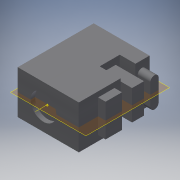
# Autodesk Inventor part: 00_RGB_Laser_Laserlands
Saved by Autodesk Inventor 2019.4 (Build 234330000, 330)
## iProperties
Created: 2021-09-30
Part Number: 00_RGB_Laser_Laserlands
Material: Generic
Document SubType Name: Modeling
Designer: diederichbenedict
Density: 1 g/cm^3
Appearance: Light Gray
Author: diederichbenedict
Autodesk Inventor part; units mm, degrees
ref_plane "YZ Plane" through (0, 0, 0) normal (1, 0, 0) x (0, 1, 0)
ref_plane "XZ Plane" through (0, 0, 0) normal (0, 1, 0) x (-1, 0, 0)
ref_plane "XY Plane" through (0, 0, 0) normal (0, 0, 1) x (1, 0, 0)
sketch "Sketch1" plane through (0, 0, 0) normal (0, 1, 0) x (-1, 0, 0)
  line L0 (0, 0) -> (41, 0)
  line L1 (0, 0) -> (41, 0) construction
  line L2 (41, 0) -> (41, -51)
  line L3 (41, -51) -> (3.5, -51)
  line L4 (3.5, -51) -> (3.5, -41.5)
  line L5 (3.5, -41.5) -> (14, -41.5)
  line L6 (14, -41.5) -> (14, -28)
  line L7 (14, -28) -> (0, -28)
  line L8 (0, -28) -> (0, 0)
  dimension "d0" = 41
  dimension "d1" = 0
  dimension "d2" = 51
  dimension "d3" = 90
  dimension "d4" = 37.5
  dimension "d5" = 90
  dimension "d6" = 9.5
  dimension "d7" = 90
  dimension "d8" = 10.5
  dimension "d9" = 13.5
  dimension "d10" = 90
  constraints: 18 end point, 7 perpendicular, 2 horizontal, 1 collinear
  measures "d0" distance of L0.start L0.end
  measures "d1" distance between parallel lines of L0 L1
  measures "d2" distance of L0.end L2.end
  measures "d3" angle of L0 L2
  measures "d4" distance of L2.end L3.end
  measures "d5" angle of L2 L3
  measures "d6" distance of L3.end L4.end
  measures "d7" angle of L3 L4
  measures "d8" distance of L4.end L5.end
  measures "d9" distance of L5.end L6.end
  measures "d10" angle of L6 L5
extrude "Extrusion1" add sketch "Sketch1" along normal blind 29
sketch "Sketch2" plane through (-41, 0, 0) normal (0, 0, 1) x (1, 0, 0)
  line L0 (41, 0) -> (0, 0) projected
  line L1 (41, 0) -> (41, 29) projected
  line L2 (0, 29) -> (41, 29) projected
  line L3 (0, 0) -> (0, 29) projected
  circle A0 centre (17.25, 14.5) radius 8.625
  dimension "d13" = 17.25
  dimension "d14" = 17.25
  dimension "d15" = 14.5
  constraints: 1 centre point
  measures "d13" diameter of A0
  measures "d14" distance from line of A0.centre L3
  measures "d15" distance from line of A0.centre L2
extrude "Extrusion2" cut sketch "Sketch2" against normal blind 3 contours A0
sketch "Sketch3" plane through (-14, 0, -28) normal (1, 0, 0) x (0, 0, -1)
  line L0 (13.5, 0) -> (0, 0) projected
  line L1 (13.5, 0) -> (13.5, 29) projected
  line L2 (0, 29) -> (13.5, 29) projected
  line L3 (0, 0) -> (0, 29) projected
  line L4 (0, 0) -> (-28, 0) projected
  line L5 (0, 0) -> (0, 29) projected
  line L6 (-28, 29) -> (0, 29) projected
  line L7 (-28, 0) -> (-28, 29) projected
  line L8 (23, 0) -> (13.5, 0) projected
  line L9 (23, 0) -> (23, 29) projected
  line L10 (13.5, 29) -> (23, 29) projected
  line L11 (13.5, 0) -> (13.5, 29) projected
  line L12 (2.7351, 24.5) -> (10.7649, 24.5)
  line L13 (10.7649, 24.5) -> (10.7649, 4.5)
  line L14 (10.7649, 4.5) -> (2.7351, 4.5)
  line L15 (2.7351, 4.5) -> (2.7351, 24.5)
  line L16 (2.7351, 24.5) -> (10.7649, 4.5) construction
  line L17 (10.7649, 24.5) -> (2.7351, 4.5) construction
  line L18 (-15.0444, 25.4539) -> (-4.0444, 25.4539)
  line L19 (-4.0444, 25.4539) -> (-4.0444, 3.5461)
  line L20 (-4.0444, 3.5461) -> (-15.0444, 3.5461)
  line L21 (-15.0444, 3.5461) -> (-15.0444, 25.4539)
  line L22 (-15.0444, 25.4539) -> (-4.0444, 3.5461) construction
  line L23 (-4.0444, 25.4539) -> (-15.0444, 3.5461) construction
  line L24 (17.7718, 7.3132) -> (17.7718, 21.6868) construction
  line L25 (20.5552, 7.3132) -> (20.5552, 21.6868)
  line L26 (14.9884, 21.6868) -> (14.9884, 7.3132)
  arc A0 (14.9884, 7.3132) -> (20.5552, 7.3132) centre (17.7718, 7.3132) ccw
  arc A1 (20.5552, 21.6868) -> (14.9884, 21.6868) centre (17.7718, 21.6868) ccw
  point P0 (6.75, 14.5)
  point P1 (-9.5444, 14.5)
  point P2 (17.7718, 14.5)
  dimension "d18" = 20
  dimension "d19" = 11
  constraints: 32 end point, 5 midpoint, 5 parallel, 4 point on circle, 4 tangent, 2 centre point, 2 horizontal, 2 perpendicular, 1 vertical
  measures "d18" distance of L12.end L13.end
  measures "d19" distance of L19.end L20.end
extrude "Extrusion3" add sketch "Sketch3" along normal blind 19 contours L12 L13 L14 L15 | L18 L19 L20 L21 | A0 L26 A1 L25
ref_plane "Work Plane1" through (-23.75, 14.5, -3) normal (0, 1, 0) x (1, 0, 0)
body "Solid1"
